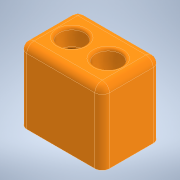
# Autodesk Inventor part: proxima_case
Saved by Autodesk Inventor 2021 (Build 250183000, 183)
## iProperties
Created: 2021-08-02
Part Number: proxima_case
Material: Generic
Document SubType Name: Modeling
Designer: ermoz
Density: 1 g/cm^3
Appearance: Default
Author: ermoz
Autodesk Inventor part; units mm, degrees
ref_plane "YZ Plane" through (0, 0, 0) normal (1, 0, 0) x (0, 1, 0)
ref_plane "XZ Plane" through (0, 0, 0) normal (0, 1, 0) x (-1, 0, 0)
ref_plane "XY Plane" through (0, 0, 0) normal (0, 0, 1) x (1, 0, 0)
sketch "Sketch1" plane through (0, 0, 0) normal (0, 1, 0) x (-1, 0, 0)
  line L0 (-7.6, 5.1) -> (7.6, 5.1)
  line L1 (7.6, 5.1) -> (7.6, -5.1)
  line L2 (7.6, -5.1) -> (-7.6, -5.1)
  line L3 (-7.6, -5.1) -> (-7.6, 5.1)
  line L4 (-7.6, 5.1) -> (7.6, -5.1) construction
  line L5 (7.6, 5.1) -> (-7.6, -5.1) construction
  line L6 (-8.5, 6) -> (8.5, 6)
  line L7 (8.5, 6) -> (8.5, -6)
  line L8 (8.5, -6) -> (-8.5, -6)
  line L9 (-8.5, -6) -> (-8.5, 6)
  line L10 (-8.5, 6) -> (8.5, -6) construction
  line L11 (8.5, 6) -> (-8.5, -6) construction
  point P0 (0, 0)
  dimension "d0" = 15.2
  dimension "d1" = 10.2
  dimension "d2" = 17
  dimension "d3" = 12
  constraints: 24 end point, 4 midpoint, 4 parallel, 2 horizontal, 2 perpendicular
  measures "d0" distance of L1.end L2.end
  measures "d1" distance of L0.end L1.end
  measures "d2" distance of L7.end L8.end
  measures "d3" distance of L6.end L7.end
extrude "Extrusion1" add sketch "Sketch1" along normal blind 15
sketch "Sketch2" plane through (0, 15, 0) normal (0, 1, 0) x (1, 0, 0)
  line L0 (8.5, 6) -> (-8.5, 6) projected
  line L1 (-8.5, 6) -> (-8.5, -6) projected
  line L2 (-8.5, -6) -> (8.5, -6) projected
  line L3 (8.5, -6) -> (8.5, 6) projected
  circle A0 centre (3.75, 0) radius 2.6
  circle A1 centre (-3.75, 0) radius 2.6
  line L4 (0, 0) -> (0, 3.4461)
  line L5 (0, 0) -> (1.0482, 0)
  dimension "d8" = 5.2
  dimension "d10" = 7.5
  constraints: 4 end point, 2 centre point, 1 equal radius, 1 horizontal, 1 horizontal alignment, 1 point on line, 1 symmetric about line, 1 vertical
  measures "d8" diameter of A0
  measures "d10" distance of A1.centre A0.centre
extrude "Extrusion2" add sketch "Sketch2" against normal blind 8
fillet "Fillet1" radius 1.5 8 edges at (-8.5, 15, 0) (0, 15, 6) (0, 15, -6) (8.5, 15, 0) (8.5, 7.5, 6) (-8.5, 7.5, 6) (-8.5, 7.5, -6) (8.5, 7.5, -6)
fillet "Fillet2" radius 0.5 2 edges at (1.15, 15, 0) (-6.35, 15, 0)
sketch "Sketch3" plane through (0, 7, 0) normal (0, -1, 0) x (1, 0, 0)
  line L0 (7.6, 5.1) -> (-7.6, 5.1) projected
  line L1 (-7.6, -5.1) -> (7.6, -5.1) projected
  line L2 (0, 5.1) -> (7.6, 5.1)
  line L3 (7.6, 5.1) -> (7.6, -5.1)
  line L4 (7.6, -5.1) -> (0, -5.1)
  line L5 (0, -5.1) -> (0, 5.1)
  line L6 (0, 5.1) -> (-7.6, 5.1)
  line L7 (-7.6, 5.1) -> (-7.6, -5.1)
  line L8 (-7.6, -5.1) -> (0, -5.1)
  line L9 (0, -5.1) -> (0, 5.1)
  point P0 (0, 0)
  point P1 (-7.6, 5.1)
  constraints: 16 end point, 4 parallel, 2 horizontal, 2 perpendicular, 1 midpoint
extrude "Extrusion3" cut sketch "Sketch3" against normal blind 4 contours L5 L1 L7 L0
fillet "Fillet3" radius 0.5 15 edges at (7.6, 3.5, -5.1) (-7.6, 5.5, -5.1) (-7.6, 5.5, 5.1) (7.6, 3.5, 5.1) (1.15, 7, 0) (-6.35, 11, 0) (-3.8, 11, -5.1) (-7.6, 11, 0) (0, 9, -5.1) (0, 11, 0) (3.8, 7, -5.1) (7.6, 7, 0) (3.8, 7, 5.1) (0, 9, 5.1) (-3.8, 11, 5.1)
sketch "Sketch4" plane through (0, 11, 0) normal (0, -1, 0) x (1, 0, 0)
  line L0 (-7.1, -5.1) -> (-0.5, -5.1) projected
  line L1 (-7.6, 5.1) -> (-6.6, 5.1)
  line L2 (-6.6, 5.1) -> (-6.6, -5.1)
  line L3 (-6.6, -5.1) -> (-7.6, -5.1)
  line L4 (-7.6, -5.1) -> (-7.6, 5.1)
  line L5 (-7.1, -5.1) -> (7.1, -5.1) projected
  line L6 (7.5652, 5.1) -> (6.4381, 5.1)
  line L7 (6.4381, 5.1) -> (6.4381, -5.1)
  line L8 (6.4381, -5.1) -> (7.5652, -5.1)
  line L9 (7.5652, -5.1) -> (7.5652, 5.1)
  point P0 (0, 0)
  dimension "d16" = 1
  constraints: 16 end point, 4 parallel, 2 horizontal, 2 perpendicular, 2 point on line
  measures "d16" distance of L2.end L3.end
extrude "Extrusion4" add sketch "Sketch4" along normal blind 7.4
body "Solid1"
